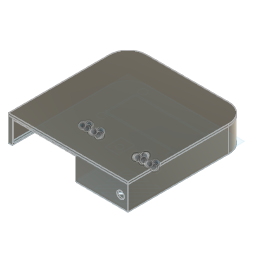
Controlador modelo 3d (sujeto a cambios) (Autodesk Fusion 360 design; units mm, degrees)
Autodesk Fusion 360 part; units mm, degrees
note: some values were not read from the file. Chosen so that the rebuilt part matches the saved one: which sketch regions a step uses; that a step has no effect; which face or edge a step refers to.
sketch "Sketch1" plane through (0, 0, 0) normal (0, 0, 1) x (1, 0, 0)
  line L0 (0, 0) -> (120, 0)
  line L1 (120, 0) -> (120, 120)
  line L2 (120, 120) -> (0, 120)
  line L3 (0, 120) -> (0, 0)
  line L4 (0, 120) -> (22, 120)
  line L5 (22, 120) -> (22, 110)
  line L6 (22, 110) -> (98, 110)
  line L7 (98, 110) -> (98, 84)
  line L8 (98, 84) -> (22, 84)
  line L9 (22, 84) -> (22, 110)
  line L10 (120, 45) -> (0, 45)
  line L11 (0, 45) -> (0, 0)
  line L12 (0, 0) -> (120, 0)
  line L13 (120, 0) -> (120, 45)
  line L14 (2, 118) -> (2, 2)
  line L15 (2, 2) -> (118, 2)
  line L16 (118, 2) -> (118, 118)
  line L17 (118, 118) -> (2, 118)
  dimension "d1" = 120
  dimension "d2" = 120
  dimension "d3" = 22
  dimension "d4" = 76
  dimension "d5" = 26
  dimension "d6" = -2
  constraint horizontal L0
  constraint vertical L1
  constraint horizontal L2
  constraint vertical L3
  constraint coincident L0.start L3.end
  constraint perpendicular L3 L4
  constraint perpendicular L4 L5
  constraint horizontal L6
  constraint vertical L7
  constraint horizontal L8
  constraint vertical L9
  constraint horizontal L10
  constraint vertical L11
  constraint horizontal L12
  constraint vertical L13
  constraint coincident L1 L10.start
  measures "d1" distance of L0.start L0.end
  measures "d2" distance of L0.start L2.end
  measures "d3" distance of L2.end L4.end
  measures "d4" distance of L5.end L6.end
  measures "d5" distance of L5.end L8.end
  measures "d43" distance of L10.end
  measures "d44" distance of L10.end
  measures "d181" distance of L10.end
  measures "d182" distance of L10.end
  measures "d201" distance of L10.end
  measures "d202" distance of L10.end
  measures "d203" distance of L10.end
sketch "Sketch2" plane through (0, 0, -50) normal (0, 0, -1) x (1, 0, 0)
  line L0 (118, -118) -> (2, -118)
  line L1 (2, -118) -> (2, -2)
  line L2 (2, -2) -> (118, -2)
  line L3 (118, -2) -> (118, -118)
  line L4 (0, 0) -> (0, -120)
  line L5 (0, -120) -> (120, -120)
  line L6 (120, -120) -> (120, 0)
  line L7 (120, 0) -> (0, 0)
  line L8 (0, 0) -> (120, 0)
  line L9 (120, 0) -> (120, -120)
  line L10 (120, -120) -> (0, -120)
  line L11 (0, -120) -> (0, 0)
  constraint horizontal L8
  constraint vertical L9
  constraint horizontal L10
  constraint vertical L11
  constraint coincident L5.end L6.start
  constraint coincident L4.start L7.end
sketch "Sketch3" plane through (120, 0, 0) normal (1, 0, 0) x (0, 1, 0)
  line L0 (120, 0) -> (0, 0)
  line L1 (0, 0) -> (0, -50)
  line L2 (0, -50) -> (120, -50)
  line L3 (120, -50) -> (120, 0)
  line L4 (0, -25) -> (50, -25)
  line L5 (50, -25) -> (50, 0)
  constraint midpoint L1 L4.start
  constraint perpendicular L1 L4
  constraint coincident L0 L5.end
  constraint perpendicular L0 L5
extrude "Extrude4" cut sketch "Sketch3" against normal blind 140 contours L0 L1 L4 L5
sketch "Sketch4" plane through (2, 0, 0) normal (1, 0, 0) x (0, 1, 0)
  line L0 (50, -2) -> (50, -25)
  line L1 (50, -25) -> (2, -25)
  line L2 (2, -25) -> (2, -48)
  line L3 (2, -48) -> (118, -48)
  line L4 (118, -48) -> (118, -2)
  line L5 (118, -2) -> (50, -2)
  line L6 (4, -27) -> (4, -46)
  line L7 (4, -46) -> (116, -46)
  line L8 (116, -46) -> (116, -4)
  line L9 (116, -4) -> (52, -4)
  line L10 (52, -4) -> (52, -27)
  line L11 (52, -27) -> (4, -27)
  line L12 (4, -27) -> (0, -27)
  line L13 (52, -4) -> (52, 0)
  dimension "d15" = -2
  constraint perpendicular L2 L12
  constraint perpendicular L5 L13
sketch "Sketch5" plane through (0, 0, 0) normal (0, 0, 1) x (-1, 0, 0)
  line L0 (-2, -50) -> (-118, -50)
  line L1 (-98, -84) -> (-22, -84)
  line L2 (-22, -84) -> (-22, -110)
  line L3 (-22, -110) -> (-98, -110)
  line L4 (-98, -110) -> (-98, -84)
  line L5 (-22, -110) -> (-98, -110)
  line L6 (-98, -110) -> (-98, -84)
  line L7 (-98, -84) -> (-22, -84)
  line L8 (-22, -84) -> (-22, -110)
  line L9 (-118, -50) -> (-118, -118)
  line L10 (-118, -118) -> (-2, -118)
  line L11 (-2, -118) -> (-2, -50)
  constraint horizontal L5
  constraint vertical L6
  constraint horizontal L7
  constraint vertical L8
  constraint coincident L1.start L4.end
  constraint coincident L2.end L3.start
sketch "Sketch6" plane through (0, 0, -1) normal (0, 0, 1) x (-1, 0, 0)
  line L0 (-22, -84) -> (-98, -84)
  line L1 (-98, -84) -> (-98, -110)
  line L2 (-98, -110) -> (-22, -110)
  line L3 (-22, -110) -> (-22, -84)
  line L4 (-22, -110) -> (-98, -110)
  line L5 (-98, -110) -> (-98, -84)
  line L6 (-98, -84) -> (-22, -84)
  line L7 (-22, -84) -> (-22, -110)
  line L8 (-35, -90) -> (-90, -90) construction
  line L9 (-90, -90) -> (-90, -105) construction
  line L10 (-90, -105) -> (-35, -105) construction
  line L11 (-35, -105) -> (-35, -90) construction
  dimension "d22" = 10
  constraint horizontal L4
  constraint vertical L5
  constraint horizontal L6
  constraint vertical L7
  constraint coincident L0.end L1.start
  constraint coincident L2.end L3.start
sketch "Sketch7" plane through (0, 0, 0) normal (0, 0, 1) x (-1, 0, 0)
  line L0 (-2, -50) -> (-118, -50)
  line L1 (-98, -84) -> (-22, -84)
  line L2 (-22, -84) -> (-22, -110)
  line L3 (-22, -110) -> (-98, -110)
  line L4 (-98, -110) -> (-98, -84)
  line L5 (-122, -120) -> (-2, -120)
  line L6 (-2, -120) -> (-2, -50)
  line L7 (-2, -50) -> (-122, -50)
  line L8 (-122, -50) -> (-122, -120)
  line L9 (-60, -79.6486) -> (-22, -79.6486)
  line L10 (-22, -79.6486) -> (-98, -79.6486)
  line L11 (-98, -79.6486) -> (-98, -69.6486)
  line L12 (-22, -69.6486) -> (-22, -79.6486)
  line L13 (-22, -79.6486) -> (-98, -79.6486)
  line L14 (-98, -79.6486) -> (-98, -67.6486)
  line L15 (-98, -67.6486) -> (-22, -67.6486)
  line L16 (-22, -67.6486) -> (-22, -79.6486)
  line L17 (-22, -79.6486) -> (-26, -79.6486)
  line L18 (-26, -79.6486) -> (-38, -79.6486)
  line L19 (-38, -67.6486) -> (-26, -67.6486)
  line L20 (-38, -67.6486) -> (-43, -67.6486)
  line L21 (-43, -67.6486) -> (-55, -67.6486)
  line L22 (-55, -79.6486) -> (-43, -79.6486)
  line L23 (-55, -67.6486) -> (-60, -67.6486)
  line L24 (-60, -67.6486) -> (-72, -67.6486)
  line L25 (-72, -79.6486) -> (-60, -79.6486)
  line L26 (-22, -79.6486) -> (-30, -79.6486)
  line L27 (-30, -79.6486) -> (-42, -79.6486)
  line L28 (-42, -79.6486) -> (-42, -67.6486)
  line L29 (-42, -67.6486) -> (-30, -67.6486)
  line L30 (-30, -67.6486) -> (-30, -79.6486)
  line L31 (-42, -67.6486) -> (-46, -67.6486)
  line L32 (-46, -67.6486) -> (-58, -67.6486)
  line L33 (-58, -67.6486) -> (-58, -79.6486)
  line L34 (-58, -79.6486) -> (-46, -79.6486)
  line L35 (-46, -79.6486) -> (-46, -67.6486)
  line L36 (-58, -79.6486) -> (-62, -79.6486)
  line L37 (-62, -79.6486) -> (-74, -79.6486)
  line L38 (-74, -79.6486) -> (-74, -67.6486)
  line L39 (-74, -67.6486) -> (-62, -67.6486)
  line L40 (-62, -67.6486) -> (-62, -79.6486)
  line L41 (-74, -67.6486) -> (-78, -67.6486)
  line L42 (-78, -67.6486) -> (-90, -67.6486)
  line L43 (-90, -67.6486) -> (-90, -79.6486)
  line L44 (-90, -79.6486) -> (-78, -79.6486)
  line L45 (-78, -79.6486) -> (-78, -67.6486)
  circle A0 centre (-36, -73.6486) radius 6
  circle A1 centre (-52, -73.6486) radius 6
  circle A2 centre (-68, -73.6486) radius 6
  circle A3 centre (-84, -73.6486) radius 6
  line L46 (-118, -50) -> (-118, -118)
  line L47 (-118, -118) -> (-2, -118)
  line L48 (-2, -118) -> (-2, -50)
  dimension "d27" = 10
  dimension "d28" = 12
  dimension "d29" = 12
  dimension "d30" = 12
  dimension "d31" = 12
  dimension "d32" = 12
  dimension "d33" = 5
  dimension "d34" = 12
  dimension "d35" = 12
  dimension "d36" = 8
  dimension "d37" = 12
  dimension "d38" = 12
  dimension "d39" = 4
  dimension "d40" = 12
  dimension "d41" = 12
  dimension "d42" = 4
  dimension "d43" = 12
  dimension "d44" = 12
  dimension "d45" = 4
  dimension "d46" = 12
  dimension "d47" = 12
  dimension "d48" = 6
  dimension "d49" = 6
  dimension "d50" = 6
  dimension "d51" = 6
  constraint horizontal L5
  constraint vertical L6
  constraint horizontal L7
  constraint vertical L8
  constraint coincident L0.start L6.end
  constraint parallel L1 L9
  constraint horizontal L10
  constraint vertical L11
  constraint vertical L12
  constraint horizontal L13
  constraint vertical L14
  constraint horizontal L15
  constraint vertical L16
  constraint coincident L9 L17.end
  constraint perpendicular L16 L17
  constraint horizontal L18
  constraint horizontal L19
  constraint coincident L15 L20.end
  constraint horizontal L21
  constraint horizontal L22
  constraint horizontal L24
  constraint horizontal L25
  constraint perpendicular L12 L26
  constraint horizontal L27
  constraint vertical L28
  constraint horizontal L29
  constraint vertical L30
  constraint perpendicular L28 L31
  constraint horizontal L32
  constraint vertical L33
  constraint horizontal L34
  constraint vertical L35
  constraint perpendicular L33 L36
  constraint horizontal L37
  constraint vertical L38
  constraint horizontal L39
  constraint vertical L40
  constraint perpendicular L38 L41
  constraint horizontal L42
  constraint vertical L43
  constraint horizontal L44
  constraint vertical L45
  constraint tangent L30 A0
  constraint tangent L15 A0
  constraint tangent L15 A1
  constraint tangent L35 A1
  constraint tangent L15 A2
  constraint tangent L40 A2
  constraint tangent L15 A3
  constraint tangent L45 A3
  measures "d27" distance of L9.end L12.start
  measures "d28" distance of L9.end L15.end
  measures "d29" distance of L17.end L18.end
  measures "d30" distance of L17.end L19.end
  measures "d31" distance of L20.end L21.end
  measures "d32" distance of L20.end L22.end
  measures "d33" distance of L21.end L23.end
  measures "d34" distance of L23.end L24.end
  measures "d35" distance of L23.end L9.start
  measures "d36" distance of L9.end L26.end
  measures "d37" distance of L26.end L27.end
  measures "d38" distance of L26.end L29.end
  measures "d39" distance of L28.end L31.end
  measures "d40" distance of L31.end L32.end
  measures "d41" distance of L31.end L34.end
  measures "d42" distance of L33.end L36.end
  measures "d43" distance of L36.end L37.end
  measures "d44" distance of L36.end L39.end
  measures "d45" distance of L38.end L41.end
  measures "d46" distance of L41.end L42.end
  measures "d47" distance of L41.end L44.end
  measures "d48" radius of A0
  measures "d49" radius of A1
  measures "d50" radius of A2
  measures "d51" radius of A3
sketch "Sketch8" plane through (0, 0, -3) normal (0, 0, -1) x (1, 0, 0)
  circle A0 centre (84, -73.6486) radius 6
  line L0 (84, -73.6486) -> (84, -67.6486)
  line L1 (84, -67.6486) -> (90, -67.6486)
  line L2 (90, -67.6486) -> (30, -67.6486)
  line L3 (30, -67.6486) -> (30, -79.6486)
  line L4 (30, -79.6486) -> (90, -79.6486)
  line L5 (90, -79.6486) -> (90, -67.6486)
  dimension "d60" = 12
  constraint coincident A0.centre L0.start
  constraint coincident A0 L0.end
  constraint vertical L0
  constraint tangent A0 L1
  constraint horizontal L2
  constraint vertical L3
  constraint horizontal L4
  constraint vertical L5
  measures "d60" distance of L1.end L4.end
sketch "Sketch9" plane through (0, 0, 0) normal (0, 0, 1) x (-1, 0, 0)
  circle A0 centre (-68, -73.6486) radius 6
  circle A1 centre (-52, -73.6486) radius 6
  circle A2 centre (-84, -73.6486) radius 6
  circle A3 centre (-36, -73.6486) radius 6
  line L0 (-2, -50) -> (-118, -50)
  line L1 (-98, -84) -> (-22, -84)
  line L2 (-22, -84) -> (-22, -110)
  line L3 (-22, -110) -> (-98, -110)
  line L4 (-98, -110) -> (-98, -84)
  line L5 (-36, -73.6486) -> (-36, -67.6486)
  line L6 (-36, -67.6486) -> (-36, -65.6486)
  line L7 (-36, -65.6486) -> (-30, -65.6486)
  line L8 (-30, -65.6486) -> (-90, -65.6486)
  line L9 (-90, -65.6486) -> (-90, -60.6486)
  line L10 (-90, -60.6486) -> (-30, -60.6486)
  line L11 (-30, -60.6486) -> (-30, -65.6486)
  line L12 (-30, -65.6486) -> (-42, -65.6486)
  line L13 (-42, -65.6486) -> (-42, -60.6486)
  line L14 (-42, -60.6486) -> (-30, -60.6486)
  line L15 (-30, -60.6486) -> (-30, -65.6486)
  line L16 (-90, -65.6486) -> (-78, -65.6486)
  line L17 (-78, -65.6486) -> (-78, -60.6486)
  line L18 (-78, -60.6486) -> (-90, -60.6486)
  line L19 (-90, -60.6486) -> (-90, -65.6486)
  line L20 (-78, -65.6486) -> (-74, -65.6486)
  line L21 (-42, -65.6486) -> (-46, -65.6486)
  line L22 (-46, -65.6486) -> (-58, -65.6486)
  line L23 (-58, -65.6486) -> (-58, -60.6486)
  line L24 (-58, -60.6486) -> (-46, -60.6486)
  line L25 (-46, -60.6486) -> (-46, -65.6486)
  line L26 (-74, -65.6486) -> (-62, -65.6486)
  line L27 (-62, -65.6486) -> (-62, -60.6486)
  line L28 (-62, -60.6486) -> (-74, -60.6486)
  line L29 (-74, -60.6486) -> (-74, -65.6486)
  line L30 (-36, -65.6486) -> (-33, -65.6486)
  line L31 (-33.5, -69.1486) -> (-33.5, -57.1486) construction
  line L32 (-33.5, -57.1486) -> (-38.5, -57.1486) construction
  line L33 (-38.5, -57.1486) -> (-38.5, -69.1486) construction
  line L34 (-38.5, -69.1486) -> (-33.5, -69.1486) construction
  line L35 (-55.1376, -57.1486) -> (-55.1376, -69.1486) construction
  line L36 (-55.1376, -69.1486) -> (-50.1376, -69.1486) construction
  line L37 (-50.1376, -69.1486) -> (-50.1376, -57.1486) construction
  line L38 (-50.1376, -57.1486) -> (-55.1376, -57.1486) construction
  line L39 (-62.3188, -60.3674) -> (-74.3188, -60.3674) construction
  line L40 (-74.3188, -60.3674) -> (-74.3188, -65.3674) construction
  line L41 (-74.3188, -65.3674) -> (-62.3188, -65.3674) construction
  line L42 (-62.3188, -65.3674) -> (-62.3188, -60.3674) construction
  line L43 (-90.3188, -65.9674) -> (-78.3188, -65.9674) construction
  line L44 (-78.3188, -65.9674) -> (-78.3188, -60.9674) construction
  line L45 (-78.3188, -60.9674) -> (-90.3188, -60.9674) construction
  line L46 (-90.3188, -60.9674) -> (-90.3188, -65.9674) construction
  line L47 (-118, -50) -> (-118, -118)
  line L48 (-118, -118) -> (-2, -118)
  line L49 (-2, -118) -> (-2, -50)
  dimension "d63" = 2
  dimension "d64" = 6
  dimension "d65" = 60
  dimension "d66" = 5
  dimension "d67" = 12
  dimension "d68" = 5
  dimension "d69" = 12
  dimension "d70" = 4
  dimension "d71" = 4
  dimension "d72" = 12
  dimension "d73" = 12
  dimension "d74" = 6
  dimension "d75" = 6
  dimension "d76" = 6
  dimension "d77" = 6
  constraint coincident A3.centre L5.start
  constraint coincident A3 L5.end
  constraint vertical L5
  constraint parallel L5 L6
  constraint perpendicular L6 L7
  constraint horizontal L8
  constraint vertical L9
  constraint horizontal L10
  constraint vertical L11
  constraint horizontal L12
  constraint vertical L13
  constraint horizontal L14
  constraint vertical L15
  constraint horizontal L16
  constraint vertical L17
  constraint horizontal L18
  constraint vertical L19
  constraint perpendicular L17 L20
  constraint perpendicular L13 L21
  constraint horizontal L22
  constraint vertical L23
  constraint horizontal L24
  constraint vertical L25
  constraint horizontal L26
  constraint vertical L27
  constraint horizontal L28
  constraint vertical L29
  constraint midpoint L7 L30.end
  measures "d63" distance of L5.end L6.end
  measures "d64" distance of L6.end L7.end
  measures "d65" distance of L7.end L8.end
  measures "d66" distance of L7.end L10.end
  measures "d67" distance of L7.end L12.end
  measures "d68" distance of L7.end L10.end
  measures "d69" distance of L8.end L16.end
  measures "d70" distance of L16.end L20.end
  measures "d71" distance of L12.end L21.end
  measures "d72" distance of L21.end L22.end
  measures "d73" distance of L20.end L26.end
extrude "Extrude16" [no effect]
sketch "Sketch10" plane through (0, 0, -25) normal (0, 0, 1) x (-1, 0, 0)
  line L0 (-119, -50) -> (-117, -50)
  line L1 (-2, -48) -> (-2, -2)
  line L2 (-118, -2) -> (-118, -48)
  line L3 (-2, -2) -> (-2, 0)
  line L4 (-2, 0) -> (-2, -50)
  line L5 (-118, -2) -> (-118, 0)
  line L6 (-173, -50) -> (-133, -50)
  line L7 (-134, -30) -> (-173, -30)
  line L8 (-173, -30) -> (-173, -50)
  line L9 (-173, -30) -> (-168, -30)
  line L10 (-168, -30) -> (-158, -30)
  line L11 (-158, -30) -> (-158, -50)
  line L12 (-158, -50) -> (-168, -50)
  line L13 (-168, -50) -> (-168, -30)
  line L14 (-158, -30) -> (-156, -30)
  line L15 (-156, -30) -> (-146, -30)
  line L16 (-146, -30) -> (-146, -50)
  line L17 (-146, -50) -> (-156, -50)
  line L18 (-156, -50) -> (-156, -30)
  line L19 (-146, -30) -> (-144, -30)
  line L20 (-144, -30) -> (-134, -30)
  line L21 (-134, -30) -> (-134, -50)
  line L22 (-134, -50) -> (-144, -50)
  line L23 (-144, -50) -> (-144, -30)
  line L24 (-134, -50) -> (-128, -50)
  line L25 (-128, -50) -> (-120, -50)
  line L26 (-120, -50) -> (-120, -40)
  line L27 (-120, -40) -> (-128, -40)
  line L28 (-128, -40) -> (-128, -50)
  line L29 (-120, -50) -> (-118, -50)
  line L30 (-118, -50) -> (-110, -50)
  line L31 (-110, -50) -> (-110, -40)
  line L32 (-110, -40) -> (-118, -40)
  line L33 (-118, -40) -> (-118, -50)
  line L34 (-110, -50) -> (-108, -50)
  line L35 (-108, -50) -> (-100, -50)
  line L36 (-100, -50) -> (-100, -40)
  line L37 (-100, -40) -> (-108, -40)
  line L38 (-108, -40) -> (-108, -50)
  line L39 (-100, -50) -> (-98, -50)
  line L40 (-98, -50) -> (-90, -50)
  line L41 (-90, -50) -> (-90, -40)
  line L42 (-90, -40) -> (-98, -40)
  line L43 (-98, -40) -> (-98, -50)
  line L44 (-90, -50) -> (-88, -50)
  line L45 (-88, -50) -> (-80, -50)
  line L46 (-80, -50) -> (-80, -40)
  line L47 (-80, -40) -> (-88, -40)
  line L48 (-88, -40) -> (-88, -50)
  line L49 (-80, -50) -> (-78, -50)
  line L50 (-78, -50) -> (-70, -50)
  line L51 (-70, -50) -> (-70, -40)
  line L52 (-70, -40) -> (-78, -40)
  line L53 (-78, -40) -> (-78, -50)
  line L54 (-70, -50) -> (-68, -50)
  line L55 (-68, -50) -> (-62, -50)
  line L56 (-62, -50) -> (-62, -44)
  line L57 (-62, -44) -> (-68, -44)
  line L58 (-68, -44) -> (-68, -50)
  line L59 (-118, -48) -> (-118, -50)
  line L60 (-117, -2) -> (-119, -2)
  line L61 (-119, -2) -> (-119, -50)
  line L62 (-117, -50) -> (-117, -2)
  dimension "d85" = 5
  dimension "d86" = 10
  dimension "d87" = 8
  dimension "d88" = 2
  constraint coincident L0 L4.end
  constraint perpendicular L0 L4
  constraint horizontal L6
  constraint horizontal L7
  constraint vertical L8
  constraint coincident L0 L6.start
  constraint perpendicular L8 L9
  constraint horizontal L10
  constraint vertical L11
  constraint horizontal L12
  constraint vertical L13
  constraint coincident L6 L11.end
  constraint coincident L7 L14.end
  constraint horizontal L15
  constraint vertical L16
  constraint horizontal L17
  constraint vertical L18
  constraint coincident L6 L16.end
  constraint coincident L7 L19.end
  constraint horizontal L20
  constraint vertical L21
  constraint horizontal L22
  constraint vertical L23
  constraint coincident L0 L24.end
  constraint horizontal L25
  constraint vertical L26
  constraint horizontal L27
  constraint vertical L28
  constraint midpoint L0 L29.end
  constraint horizontal L30
  constraint vertical L31
  constraint horizontal L32
  constraint vertical L33
  constraint coincident L0 L34.end
  constraint perpendicular L31 L34
  constraint horizontal L35
  constraint vertical L36
  constraint horizontal L37
  constraint vertical L38
  constraint coincident L0 L39.end
  constraint perpendicular L36 L39
  constraint horizontal L40
  constraint vertical L41
  constraint horizontal L42
  constraint vertical L43
  constraint perpendicular L41 L44
  constraint horizontal L45
  constraint vertical L46
  constraint horizontal L47
  constraint vertical L48
  constraint coincident L0 L49.end
  constraint perpendicular L46 L49
  constraint horizontal L50
  constraint vertical L51
  constraint horizontal L52
  constraint vertical L53
  constraint coincident L0 L54.end
  constraint perpendicular L51 L54
  constraint horizontal L55
  constraint vertical L56
  constraint horizontal L57
  constraint vertical L58
  constraint coincident L0 L29.end
  constraint perpendicular L0 L59
  measures "d85" distance of L7.end L9.end
  measures "d86" distance of L19.end L7.start
  measures "d87" distance of L29.end L30.end
  measures "d88" distance of L40.end L44.end
sketch "Sketch11" plane through (0, 50, 0) normal (0, 1, 0) x (-1, 0, 0)
  line L0 (-110, -25) -> (-100, -25)
  line L1 (-100, -25) -> (-100, -15)
  line L2 (-100, -15) -> (-110, -15)
  line L3 (-110, -15) -> (-110, -25)
  line L4 (-110, -15) -> (-4, -15)
  line L5 (-4, -15) -> (-4, -25)
  line L6 (-4, -25) -> (-110, -25)
  line L7 (-110, -25) -> (-110, -15)
  constraint horizontal L4
  constraint vertical L5
  constraint horizontal L6
  constraint vertical L7
  constraint coincident L2.end L3.start
sketch "Sketch12" plane through (0, 0, 0) normal (0, 0, 1) x (-1, 0, 0)
  line L0 (-118, -2) -> (-234, -2)
  line L1 (-234, -2) -> (-234, 48)
  line L2 (-234, 48) -> (-118, 48)
  line L3 (-118, 48) -> (-118, -2)
  line L4 (-118, 0) -> (-2, 0)
  line L5 (-2, 0) -> (-2, -2)
  line L6 (-2, -2) -> (-118, -2)
  line L7 (-118, -2) -> (-118, 0)
  line L8 (-118, -2) -> (-119, -2)
  line L9 (-119, -2) -> (-119, -50)
  line L10 (-118, -50) -> (-118, -2)
  line L11 (-119, -50) -> (-118, -50)
  dimension "d95" = 2
  constraint horizontal L0
  constraint vertical L1
  constraint horizontal L2
  constraint vertical L3
  constraint coincident L0.start L3.end
  constraint horizontal L4
  constraint vertical L5
  constraint horizontal L6
  constraint vertical L7
  measures "d95" distance of L4.start L0.start
extrude "Extrude25" [no effect]
sketch "Sketch13" plane through (0, 0, 0) normal (1, 0, 0) x (0, 1, 0)
  line L0 (42, -15) -> (40, -17)
  line L1 (42, -15) -> (40, -15)
  line L2 (40, -15) -> (40, -17)
  constraint horizontal L1
  constraint perpendicular L1 L2
extrude "Extrude26" cut sketch "Sketch13" along normal blind 115
sketch "Sketch14" plane through (0, 40, 0) normal (0, -1, 0) x (1, 0, 0)
  line L0 (10, -17) -> (4, -17)
  line L1 (4, -17) -> (4, -25)
  line L2 (4, -25) -> (10, -25)
  line L3 (10, -25) -> (10, -17)
  line L4 (5, -18) -> (9, -18)
  line L5 (9, -18) -> (9, -24)
  line L6 (9, -24) -> (5, -24)
  line L7 (5, -24) -> (5, -18)
  line L8 (13, -18) -> (19, -18)
  line L9 (19, -18) -> (19, -24)
  line L10 (19, -24) -> (13, -24)
  line L11 (13, -24) -> (13, -18)
  line L12 (23, -18) -> (29, -18)
  line L13 (29, -18) -> (29, -24)
  line L14 (29, -24) -> (23, -24)
  line L15 (23, -24) -> (23, -18)
  line L16 (33, -18) -> (39, -18)
  line L17 (39, -18) -> (39, -24)
  line L18 (39, -24) -> (33, -24)
  line L19 (33, -24) -> (33, -18)
  line L20 (43, -18) -> (49, -18)
  line L21 (49, -18) -> (49, -24)
  line L22 (49, -24) -> (43, -24)
  line L23 (43, -24) -> (43, -18)
  line L24 (53, -18) -> (59, -18)
  line L25 (59, -18) -> (59, -24)
  line L26 (59, -24) -> (53, -24)
  line L27 (53, -24) -> (53, -18)
  line L28 (63, -18) -> (69, -18)
  line L29 (69, -18) -> (69, -24)
  line L30 (69, -24) -> (63, -24)
  line L31 (63, -24) -> (63, -18)
  line L32 (77, -18) -> (85, -18)
  line L33 (85, -18) -> (85, -24)
  line L34 (85, -24) -> (77, -24)
  line L35 (77, -24) -> (77, -18)
  line L36 (89, -18) -> (97, -18)
  line L37 (97, -18) -> (97, -24)
  line L38 (97, -24) -> (89, -24)
  line L39 (89, -24) -> (89, -18)
  line L40 (101, -18) -> (109, -18)
  line L41 (109, -18) -> (109, -24)
  line L42 (109, -24) -> (101, -24)
  line L43 (101, -24) -> (101, -18)
  constraint horizontal L4
  constraint vertical L5
  constraint horizontal L6
  constraint vertical L7
  constraint horizontal L8
  constraint vertical L9
  constraint horizontal L10
  constraint vertical L11
  constraint horizontal L12
  constraint vertical L13
  constraint horizontal L14
  constraint vertical L15
  constraint horizontal L16
  constraint vertical L17
  constraint horizontal L18
  constraint vertical L19
  constraint horizontal L20
  constraint vertical L21
  constraint horizontal L22
  constraint vertical L23
  constraint horizontal L24
  constraint vertical L25
  constraint horizontal L26
  constraint vertical L27
  constraint horizontal L28
  constraint vertical L29
  constraint horizontal L30
  constraint vertical L31
  constraint horizontal L32
  constraint vertical L33
  constraint horizontal L34
  constraint vertical L35
  constraint horizontal L36
  constraint vertical L37
  constraint horizontal L38
  constraint vertical L39
  constraint horizontal L40
  constraint vertical L41
  constraint horizontal L42
  constraint vertical L43
extrude "Extrude27" cut sketch "Sketch14" against normal blind 10 contours L4 L5 L6 L7 | L8 L9 L10 L11 | L12 L13 L14 L15 | L16 L17 L18 L19 | L20 L21 L22 L23 | L24 L25 L26 L27 | L28 L29 L30 L31 | L32 L33 L34 L35 | L36 L37 L38 L39 | L40 L41 L42 L43
sketch "Sketch15" plane through (0, 0, -15) normal (0, 0, 1) x (-1, 0, 0)
  line L0 (-4, -50) -> (-110, -50)
  line L1 (-110, -50) -> (-110, -54)
  line L2 (-110, -54) -> (-4, -54)
  line L3 (-4, -54) -> (-4, -50)
  circle A0 centre (-7, -45) radius 2
  circle A1 centre (-16, -45) radius 2
  circle A2 centre (-26, -45) radius 2
  circle A3 centre (-36, -45) radius 2
  circle A4 centre (-46, -45) radius 2
  circle A5 centre (-56, -45) radius 2
  circle A6 centre (-66, -45) radius 2
  circle A7 centre (-81, -45) radius 2
  circle A8 centre (-93, -45) radius 2
  circle A9 centre (-105, -45) radius 2
extrude "Extrude28" cut sketch "Sketch15" against normal blind 2 contours A0 | A1 | A2 | A3 | A4 | A5 | A6 | A7 | A8 | A9
sketch "Sketch16" plane through (0, 0, -17) normal (0, 0, 1) x (-1, 0, 0)
  circle A0 centre (-105, -45) radius 1.7589
  line L0 (-104.8, -45.2) -> (-104.8, -46.7475)
  line L1 (-104.8, -44.8) -> (-104.8, -43.2525)
  line L2 (-105.2, -45.2) -> (-105.2, -46.7475)
  line L3 (-105.2, -44.8) -> (-105.2, -43.2525)
  line L4 (-105.2, -45.2) -> (-106.7475, -45.2)
  line L5 (-105.2, -44.8) -> (-106.7475, -44.8)
  line L6 (-104.8, -45.2) -> (-103.2525, -45.2)
  line L7 (-105.2, -43.2525) -> (-105.2, -44.8)
  line L8 (-105.2, -45.2) -> (-105.2, -46.7475)
  line L9 (-106.7589, -44.8) -> (-105.2, -44.8)
  line L10 (-104.8, -44.8) -> (-103.2525, -44.8)
  line L11 (-104.8, -46.7475) -> (-104.8, -45.2)
  line L12 (-104.8, -44.8) -> (-104.8, -43.2525)
  line L13 (-8.7321, -44) -> (-5.2679, -44)
  arc A1 (-5.2679, -44) -> (-8.7321, -44) centre (-7, -45) ccw
  constraint vertical L11
  constraint vertical L7
  constraint horizontal L9
  constraint collinear L7 L8
  constraint collinear L9 L10
  constraint collinear L11 L12
  constraint coincident A0 L4.end
  constraint coincident A0 L5.end
  constraint coincident A0 L3.end
  constraint coincident A0 L1.end
  constraint coincident A0 L10.end
  constraint coincident A0 L6.end
  constraint coincident A0 L0.end
  constraint coincident A0 L2.end
sketch "Sketch17" plane through (0, 0, 0) normal (0, 0, 1) x (1, 0, 0)
  line L0 (0, 0) -> (98, 0)
  line L1 (98, 0) -> (98, 40)
  line L2 (98, 40) -> (0, 40)
  line L3 (0, 40) -> (0, 0)
  line L4 (0, 0) -> (0, -30)
  circle A0 centre (4, -30) radius 4
  circle A1 centre (49, -30) radius 4
  circle A2 centre (94, -30) radius 4
  circle A3 centre (49, -30) radius 4
  circle A4 centre (4, -30) radius 4
  line L5 (0, 0) -> (0, -30)
  circle A5 centre (94, -30) radius 4
  line L6 (0, -30) -> (98, -30)
  line L7 (26.5, -30) -> (19.5, -30)
  line L8 (71.5, -30) -> (78.5, -30)
  circle A6 centre (19.5, -30) radius 4
  circle A7 centre (78.5, -30) radius 4
  circle A8 centre (49, -30) radius 15
  line L9 (-30, 60) -> (128, 60)
  line L10 (128, 60) -> (128, -70)
  line L11 (128, -70) -> (-30, -70)
  line L12 (-30, -70) -> (-30, 60)
  line L13 (-30, -70) -> (128, -70)
  line L14 (128, -70) -> (128, -100)
  line L15 (128, -100) -> (-30, -100)
  line L16 (-30, -100) -> (-30, -70)
  line L17 (-30, 60) -> (128, 60)
  line L18 (128, 60) -> (128, -100)
  line L19 (128, -100) -> (-30, -100)
  line L20 (-30, -100) -> (-30, 60)
  line L21 (-25, -100) -> (-25, -95)
  line L22 (-25, -95) -> (-25, -70)
  line L23 (-25, -70) -> (-25, -100)
  line L24 (-25, -70) -> (30, -70)
  line L25 (-25, -70) -> (50, -70)
  line L26 (-25, -70) -> (70, -70)
  line L27 (-25, -70) -> (60, -70)
  line L28 (60, -70) -> (60, -100)
  dimension "d130" = 98
  dimension "d131" = 40
  dimension "d132" = 8
  dimension "d135" = 90
  dimension "d136" = 0
  dimension "d139" = 90
  dimension "d140" = 0
  dimension "d141" = 8
  dimension "d142" = 7
  dimension "d143" = 7
  dimension "d144" = 8
  dimension "d145" = 8
  dimension "d146" = 30
  dimension "d147" = 158
  dimension "d148" = 158
  dimension "d149" = 30
  dimension "d150" = 55
  dimension "d151" = 75
  dimension "d152" = 85
  dimension "d153" = 160
  dimension "d154" = 158
  constraint horizontal L0
  constraint vertical L1
  constraint horizontal L2
  constraint vertical L3
  constraint coincident L0.start L3.end
  constraint perpendicular L0 L4
  constraint coincident L4.end A0
  constraint coincident L4.end A4
  constraint coincident A2 L6.end
  constraint perpendicular L5 L6
  constraint parallel L6 L7
  constraint parallel L6 L8
  constraint coincident L7.end A6.centre
  constraint coincident L8.end A7.centre
  constraint concentric A1 A8
  constraint horizontal L9
  constraint vertical L10
  constraint horizontal L11
  constraint vertical L12
  constraint horizontal L13
  constraint vertical L14
  constraint horizontal L15
  constraint vertical L16
  constraint horizontal L17
  constraint vertical L18
  constraint horizontal L19
  constraint vertical L20
  constraint coincident L15 L21.start
  constraint perpendicular L15 L21
  constraint coincident L11 L22.end
  constraint perpendicular L11 L22
  constraint perpendicular L22 L24
  constraint perpendicular L22 L25
  constraint coincident L13 L26.end
  constraint perpendicular L22 L27
  constraint coincident L15 L28.end
  constraint perpendicular L15 L28
  measures "d130" distance of L0.start L0.end
  measures "d131" distance of L0.start L2.end
  measures "d132" diameter of A0
  measures "d141" diameter of A4
  measures "d142" distance of L7.start L7.end
  measures "d143" distance of L8.start L8.end
  measures "d144" diameter of A6
  measures "d145" diameter of A7
  measures "d146" diameter of A8
  measures "d147" distance of L9.start L9.end
  measures "d148" distance of L11.end L10.end
  measures "d149" distance of L11.end L15.end
  measures "d150" distance of L22.end L24.end
  measures "d151" distance of L22.end L25.end
  measures "d152" distance of L22.end L27.end
  measures "d153" distance of L9.start L15.end
  measures "d154" distance of L14.end L15.end
sketch "Sketch18" plane through (0, 0, 0) normal (0, 0, 1) x (1, 0, 0)
  line L0 (-30, 60) -> (130, 60)
  line L1 (130, 60) -> (130, -100)
  line L2 (130, -100) -> (-30, -100)
  line L3 (-30, -100) -> (-30, 60)
  line L4 (128, -98) -> (-28, -98)
  line L5 (-28, -98) -> (-28, 58)
  line L6 (-28, 58) -> (128, 58)
  line L7 (128, 58) -> (128, -98)
  dimension "d155" = 2
  constraint horizontal L0
  constraint vertical L1
  constraint horizontal L2
  constraint vertical L3
extrude "Extrude32" add sketch "Sketch18" along normal blind 2 separate body contours L4 L5 L6 L7 makes body 1
extrude "Extrude33" add sketch "Sketch18" along normal blind 32 bodies 1
extrude "Extrude34" cut sketch "Sketch17" along normal blind 30 contours L0 L1 L2 L3 | A0 A4 L6 | A0 A4 L6 | A1 A3 L6 | A1 A3 L6 | A2 A5 L6 | A2 A5 L6 | L6 L7 A6 | L6 L7 A6 | L6 L8 A7 | L6 L8 A7 | L11 L13 L15 L19 L21 L22 L23 L24 L25 L26 L27 L28 bodies 1
sketch "Sketch19" plane through (0, 0, 2) normal (0, 0, 1) x (-1, 0, 0)
  line L0 (-60, 70) -> (-60, 98)
  line L1 (-60, 98) -> (-128, 98)
  line L2 (-128, 98) -> (-128, -58)
  line L3 (-128, -58) -> (28, -58)
  line L4 (28, -58) -> (28, 98)
  line L5 (28, 98) -> (25, 98)
  line L6 (25, 98) -> (25, 70)
  line L7 (25, 70) -> (-60, 70)
  line L8 (0, -40) -> (-98, -40)
  line L9 (-98, -40) -> (-98, 0)
  line L10 (-98, 0) -> (0, 0)
  line L11 (0, 0) -> (0, -40)
  circle A0 centre (-4, 30) radius 4
  circle A1 centre (-94, 30) radius 4
  circle A2 centre (-49, 30) radius 4
  circle A3 centre (-19.5, 30) radius 4
  circle A4 centre (-78.5, 30) radius 4
  circle A5 centre (-2.5, -47.5) radius 2.5
  arc A6 (-95.5, -50) -> (-95.5, -45) centre (-95.5, -47.5) ccw
  circle A7 centre (-95.5, -47.5) radius 2.5
  circle A8 centre (-95.5, -47.5) radius 5
  arc A9 (-98, 7.5) -> (-95.5, 10) centre (-95.5, 7.5) ccw
  circle A10 centre (-95.5, 7.5) radius 2.5
  arc A11 (-2.5, 10) -> (-2.5, 5) centre (-2.5, 7.5) ccw
  circle A12 centre (-2.5, 7.5) radius 2.5
  circle A13 centre (-2.5, 7.5) radius 5
  circle A14 centre (-95.5, 7.5) radius 5
  circle A15 centre (-2.5, -47.5) radius 5
  dimension "d165" = 10
  dimension "d166" = 10
  dimension "d167" = 10
  dimension "d168" = 10
  constraint concentric A6 A7
  constraint coincident A6.end A7
  constraint concentric A6 A8
  constraint concentric A9 A10
  constraint coincident A9.end A10
  constraint concentric A11 A12
  constraint coincident A11.end A12
  constraint concentric A11 A13
  constraint concentric A9 A14
  constraint concentric A5 A15
  measures "d165" diameter of A8
  measures "d166" diameter of A13
  measures "d167" diameter of A14
  measures "d168" diameter of A15
extrude "Extrude35" add sketch "Sketch19" along normal blind 8 contours A8 | A13 | A14 | A15 bodies 1
sketch "Sketch20" plane through (0, 0, 2) normal (0, 0, 1) x (-1, 0, 0)
  circle A0 centre (-2.5, -47.5) radius 5
  circle A1 centre (-95.5, -47.5) radius 5
  line L0 (-60, 70) -> (-60, 98)
  line L1 (-60, 98) -> (-128, 98)
  line L2 (-128, 98) -> (-128, -58)
  line L3 (-128, -58) -> (28, -58)
  line L4 (28, -58) -> (28, 98)
  line L5 (28, 98) -> (25, 98)
  line L6 (25, 98) -> (25, 70)
  line L7 (25, 70) -> (-60, 70)
  line L8 (0, -40) -> (-98, -40)
  line L9 (-98, -40) -> (-98, 0)
  line L10 (-98, 0) -> (0, 0)
  line L11 (0, 0) -> (0, -40)
  circle A2 centre (-4, 30) radius 4
  circle A3 centre (-94, 30) radius 4
  circle A4 centre (-49, 30) radius 4
  circle A5 centre (-19.5, 30) radius 4
  circle A6 centre (-78.5, 30) radius 4
  circle A7 centre (-95.5, 7.5) radius 5
  circle A8 centre (-2.5, 7.5) radius 5
  line L12 (-49, 20) -> (-57, 20)
  line L13 (-57, 20) -> (-41, 20)
  line L14 (-41, 46) -> (-57, 46)
  line L15 (-49, 20) -> (-41, 20)
  line L16 (-41, 20) -> (-41, 46)
  line L17 (-41, 20) -> (-59, 20)
  line L18 (-59, 20) -> (-59, 46)
  line L19 (-59, 46) -> (-41, 46)
  line L20 (-41, 46) -> (-41, 20)
  line L21 (-49, 22) -> (-43, 22)
  line L22 (-43, 22) -> (-49, 22)
  line L23 (-55, 24) -> (-55, 36)
  line L24 (-55, 36) -> (-43, 36)
  line L25 (-43, 36) -> (-43, 24)
  line L26 (-43, 24) -> (-55, 24)
  line L27 (-55, 24) -> (-55, 36)
  line L28 (-43, 22) -> (-55, 22)
  line L29 (-55, 22) -> (-55, 38)
  line L30 (-55, 38) -> (-43, 38)
  line L31 (-43, 38) -> (-43, 22)
  line L32 (-55, 22) -> (-55, 20)
  line L33 (-55, 20) -> (-57, 20)
  line L34 (-57, 20) -> (-57, 23)
  line L35 (-55, 38) -> (-55, 46)
  line L36 (-57, 46) -> (-57, 41)
  circle A9 centre (-57, 39) radius 2
  circle A10 centre (-57, 25) radius 2
  line L37 (-41, 46) -> (-59, 46)
  line L38 (-59, 46) -> (-59, 42)
  line L39 (-59, 42) -> (-41, 42)
  line L40 (-41, 42) -> (-41, 46)
  dimension "d173" = 10
  dimension "d174" = 8
  dimension "d176" = 26
  dimension "d177" = 18
  dimension "d178" = 6
  dimension "d181" = 12
  dimension "d182" = 12
  dimension "d183" = 3
  dimension "d184" = 5
  dimension "d185" = 4
  constraint horizontal L13
  constraint horizontal L14
  constraint perpendicular L14 L16
  constraint horizontal L17
  constraint vertical L18
  constraint horizontal L19
  constraint vertical L20
  constraint perpendicular L16 L21
  constraint parallel L21 L22
  constraint horizontal L24
  constraint vertical L25
  constraint horizontal L26
  constraint vertical L27
  constraint horizontal L28
  constraint vertical L29
  constraint horizontal L30
  constraint vertical L31
  constraint coincident L13 L32.end
  constraint coincident L12 L32.end
  constraint perpendicular L13 L34
  constraint coincident L19 L35.end
  constraint coincident L14 L35.end
  constraint perpendicular L14 L36
  constraint coincident L36.end A9
  constraint coincident L34.end A10
  constraint horizontal L37
  constraint vertical L38
  constraint horizontal L39
  constraint vertical L40
  measures "d173" distance of A4.centre L12.start
  measures "d174" distance of L12.start L12.end
  measures "d176" distance of L12.end L14.end
  measures "d177" distance of L13.end L17.end
  measures "d178" distance of L21.start L21.end
  measures "d181" distance of L23.start L23.end
  measures "d182" distance of L23.end L23.start
  measures "d183" distance of L12.end L34.end
  measures "d184" distance of L14.end L36.end
  measures "d185" distance of L14.start L39.end
sketch "Sketch21" plane through (0, 0, 2) normal (0, 0, 1) x (-1, 0, 0)
  line L0 (-41, 46) -> (-59, 46)
  line L1 (-59, 46) -> (-59, 42)
  line L2 (-59, 42) -> (-41, 42)
  line L3 (-41, 42) -> (-41, 46)
  constraint horizontal L0
  constraint vertical L1
  constraint horizontal L2
  constraint vertical L3
extrude "Extrude36" add sketch "Sketch20" along normal blind 5 contours L12 L13 L15 L16 L17 L20 L21 L22 L25 L28 L30 L31 L32 L35 L39 | L12 L13 L17 L23 L27 L29 L32 L33 L34 A10 | L17 L18 L34 A10 | A10 | L35 L36 A9 L39 | L18 L23 L27 L29 L35 A9 A10 | A9 | L18 L36 A9 L39 bodies 1
sketch "Sketch22" plane through (0, 0, 2) normal (0, 0, 1) x (-1, 0, 0)
  circle A0 centre (-2.5, 7.5) radius 5
  circle A1 centre (-95.5, 7.5) radius 5
  circle A2 centre (-78.5, 30) radius 4
  circle A3 centre (-19.5, 30) radius 4
  circle A4 centre (-94, 30) radius 4
  circle A5 centre (-4, 30) radius 4
  line L0 (0, -40) -> (-98, -40)
  line L1 (-98, -40) -> (-98, 0)
  line L2 (-98, 0) -> (0, 0)
  line L3 (0, 0) -> (0, -40)
  line L4 (-60, 70) -> (-60, 98)
  line L5 (-60, 98) -> (-128, 98)
  line L6 (-128, 98) -> (-128, -58)
  line L7 (-128, -58) -> (28, -58)
  line L8 (28, -58) -> (28, 98)
  line L9 (28, 98) -> (25, 98)
  line L10 (25, 98) -> (25, 70)
  line L11 (25, 70) -> (-60, 70)
  circle A6 centre (-95.5, -47.5) radius 5
  circle A7 centre (-2.5, -47.5) radius 5
  line L12 (-59, 42) -> (-41, 42)
  line L13 (-41, 42) -> (-41, 20)
  line L14 (-41, 20) -> (-55, 20)
  line L15 (-55, 20) -> (-57, 20)
  line L16 (-57, 20) -> (-59, 20)
  line L17 (-59, 20) -> (-59, 42)
  circle A8 centre (-4, 30) radius 6
  circle A9 centre (-19.5, 30) radius 6
  circle A10 centre (-78.5, 30) radius 6
  circle A11 centre (-94, 30) radius 6
  line L18 (-3, 24.0839) -> (-3, 26.127)
  line L19 (-5, 26.127) -> (-5, 24.0839)
  line L20 (-0.1459, 31.0705) -> (1.6235, 32.092)
  line L21 (0.6235, 33.8241) -> (-1.1459, 32.8025)
  line L22 (-6.8541, 32.8025) -> (-8.6235, 33.8241)
  line L23 (-9.6235, 32.092) -> (-7.8541, 31.0705)
  line L24 (-19.5, 24) -> (-18.5, 24)
  line L25 (-18.5, 24) -> (-20.5, 24)
  line L26 (-18.5, 24) -> (-18.5, 26.127)
  line L27 (-20.5, 24) -> (-20.5, 26.127)
  line L28 (-25.1962, 32.134) -> (-23.3541, 31.0705)
  line L29 (-24.1962, 33.866) -> (-22.3541, 32.8025)
  line L30 (-14.8038, 33.866) -> (-16.6459, 32.8025)
  line L31 (-13.8038, 32.134) -> (-15.6459, 31.0705)
  line L32 (-78.5, 24) -> (-77.5, 24)
  line L33 (-77.5, 24) -> (-78.5, 24)
  line L34 (-77.5, 24) -> (-78.5, 24)
  line L35 (-77.5, 24) -> (-79.5, 24)
  line L36 (-73.8038, 33.866) -> (-75.6459, 32.8025)
  line L37 (-83.1962, 33.866) -> (-81.3541, 32.8025)
  line L38 (-84.1962, 32.134) -> (-82.3541, 31.0705)
  line L39 (-79.5, 24) -> (-79.5, 26.127)
  line L40 (-77.5, 24) -> (-77.5, 26.127)
  line L41 (-72.8038, 32.134) -> (-74.6459, 31.0705)
  line L42 (-94, 24) -> (-93, 24)
  line L43 (-93, 24) -> (-95, 24)
  line L44 (-88.3038, 32.134) -> (-90.1459, 31.0705)
  line L45 (-91.1459, 32.8025) -> (-89.3038, 33.866)
  line L46 (-98.6962, 33.866) -> (-96.8541, 32.8025)
  line L47 (-95, 24) -> (-95, 26.127)
  line L48 (-97.8541, 31.0705) -> (-99.6962, 32.134)
  line L49 (-93, 26.127) -> (-93, 24)
  dimension "d188" = 12
  dimension "d189" = 12
  dimension "d190" = 12
  dimension "d191" = 12
  dimension "d196" = 1
  dimension "d197" = 2
  dimension "d200" = 1
  dimension "d201" = 1
  dimension "d202" = 1
  dimension "d203" = 2
  dimension "d206" = 1
  constraint concentric A5 A8
  constraint concentric A3 A9
  constraint concentric A2 A10
  constraint concentric A4 A11
  constraint coincident A8 L23.start
  constraint coincident A8 L22.end
  constraint coincident A8 L19.end
  constraint coincident A8 L18.start
  constraint coincident A8 L20.end
  constraint coincident A8 L21.start
  constraint coincident A9 L24.start
  constraint perpendicular L24 L26
  constraint perpendicular L25 L27
  constraint coincident A5 L18.end
  constraint coincident A5 L19.start
  constraint coincident A5 L23.end
  constraint coincident A5 L22.start
  constraint coincident A5 L21.end
  constraint coincident A5 L20.start
  constraint coincident A3 L26.end
  constraint coincident A3 L27.end
  constraint coincident A3 L28.end
  constraint coincident A3 L29.end
  constraint coincident A3 L30.end
  constraint coincident A3 L31.end
  constraint coincident A10 L32.start
  constraint parallel L33 L34
  constraint parallel L34 L35
  constraint perpendicular L35 L39
  constraint perpendicular L34 L40
  constraint coincident A2 L39.end
  constraint coincident A2 L40.end
  constraint coincident A2 L41.end
  constraint coincident A2 L36.end
  constraint coincident A2 L37.end
  constraint coincident A2 L38.end
  constraint coincident A11 L42.start
  constraint horizontal L43
  constraint vertical L47
  constraint coincident A4 L47.end
  constraint coincident A4 L48.start
  constraint coincident A4 L49.start
  constraint coincident A4 L46.end
  constraint coincident A4 L45.start
  constraint coincident A4 L44.end
  measures "d188" diameter of A8
  measures "d189" diameter of A9
  measures "d190" diameter of A10
  measures "d191" diameter of A11
  measures "d196" distance of L24.start L24.end
  measures "d197" distance of L24.end L25.end
  measures "d200" distance of L32.start L32.end
  measures "d201" distance of L32.end L32.start
  measures "d202" distance of L32.end L32.start
  measures "d203" distance of L32.end L35.end
  measures "d206" distance of L42.start L42.end
extrude "Extrude37" add sketch "Sketch22" along normal blind 3 contours A2 A10 L40 L41 | A2 A10 L36 L41 | A2 A10 L39 L40 | A2 A10 L36 L37 | A2 A10 L38 L39 | A2 A10 L37 L38 | A3 A9 L26 L31 | A3 A9 L30 L31 | A3 A9 L26 L27 | A3 A9 L29 L30 | A3 A9 L27 L28 | A3 A9 L28 L29 | A4 A11 L44 L49 | A4 A11 L44 L45 | A4 A11 L47 L49 | A4 A11 L45 L46 | A4 A11 L47 L48 | A4 A11 L46 L48 | A5 A8 L18 L20 | A5 A8 L20 L21 | A5 A8 L18 L19 | A5 A8 L21 L22 | A5 A8 L19 L23 | A5 A8 L22 L23 bodies 1
sketch "Sketch23" plane through (0, 0, 5) normal (0, 0, 1) x (-1, 0, 0)
  circle A0 centre (-4, 30) radius 4
  circle A1 centre (-4, 30) radius 6
extrude "Extrude38" cut sketch "Sketch22" along normal blind 4 contours A2 | A2 A10 L36 L41 | A2 A10 L39 L40 | A2 A10 L37 L38 | A4 | A4 A11 L44 L45 | A4 A11 L47 L49 | A4 A11 L46 L48 bodies 1
extrude "Extrude39" cut sketch "Sketch22" along normal blind 4 contours A3 | A3 A9 L30 L31 | A3 A9 L26 L27 | A3 A9 L28 L29 | A5 | A5 A8 L20 L21 | A5 A8 L18 L19 | A5 A8 L22 L23 bodies 1
sketch "Sketch24" plane through (0, -100, 0) normal (0, -1, 0) x (1, 0, 0)
  line L0 (-25, 0) -> (-25, 30)
  line L1 (-25, 30) -> (60, 30)
  line L2 (60, 30) -> (60, 0)
  line L3 (60, 0) -> (130, 0)
  line L4 (130, 0) -> (130, 32)
  line L5 (130, 32) -> (-30, 32)
  line L6 (-30, 32) -> (-30, 0)
  line L7 (-30, 0) -> (-25, 0)
  circle A0 centre (120, 15) radius 5
extrude "Extrude40" cut sketch "Sketch24" against normal blind 26 contours A0 bodies 1
fillet "Fillet5" radius 25 4 edges at (128, 58, 17) (-28, 58, 17) (130, 60, 16) (-30, 60, 16) on bodies 1
sketch "Sketch25" plane through (0, 0, 0) normal (0, 0, -1) x (1, 0, 0)
  arc A0 (-30, -35) -> (-5, -60) centre (-5, -35) ccw
  line L0 (-5, -60) -> (105, -60)
  arc A1 (105, -60) -> (130, -35) centre (105, -35) ccw
  line L1 (130, -35) -> (130, 100)
  line L2 (130, 100) -> (60, 100)
  line L3 (60, 100) -> (60, 70)
  line L4 (60, 70) -> (-25, 70)
  line L5 (-25, 70) -> (-25, 100)
  line L6 (-25, 100) -> (-30, 100)
  line L7 (-30, 100) -> (-30, -35)
  line L8 (98, -40) -> (0, -40)
  line L9 (0, -40) -> (0, 0)
  line L10 (0, 0) -> (98, 0)
  line L11 (98, 0) -> (98, -40)
  circle A2 centre (4, 30) radius 4
  circle A3 centre (94, 30) radius 4
  circle A4 centre (49, 30) radius 4
  circle A5 centre (19.5, 30) radius 4
  circle A6 centre (78.5, 30) radius 4
  line L12 (80, 95) -> (125, 50)
  line L13 (89, 95) -> (125, 59)
  line L14 (98, 95) -> (125, 68)
  line L15 (107, 95) -> (125, 77)
  line L16 (116, 95) -> (125, 86)
  line L17 (80, 87) -> (117, 50)
  line L18 (80, 79) -> (109, 50)
  line L19 (80, 71) -> (101, 50)
  line L20 (80, 63) -> (93, 50)
  line L21 (80, 55) -> (85, 50)
  line L22 (116, 95) -> (107, 95)
  line L23 (98, 95) -> (80, 95)
  line L24 (89, 95) -> (98, 95)
  line L25 (107, 95) -> (116, 95)
  line L26 (125, 59) -> (125, 68)
  line L27 (125, 77) -> (125, 86)
  line L28 (80, 95) -> (80, 87)
  line L29 (117, 50) -> (125, 50)
  line L30 (85, 50) -> (93, 50)
  line L31 (101, 50) -> (109, 50)
  line L32 (80, 79) -> (80, 71)
  line L33 (80, 63) -> (80, 55)
  constraint horizontal L22
  constraint vertical L28
  constraint horizontal L30
  constraint vertical L26
  constraint coincident L19.end L30
  constraint coincident L17.end L30
  constraint coincident L13.start L22
  constraint coincident L14.start L22
  constraint collinear L22 L23
  constraint collinear L24 L25
  constraint collinear L26 L27
  constraint collinear L28 L32
  constraint collinear L29 L30
  constraint collinear L30 L31
  constraint collinear L32 L33
extrude "Extrude41" cut sketch "Sketch25" against normal blind 5 contours L12 L17 L28 L29 | L13 L14 L23 L24 L26 | L15 L16 L22 L25 L27 | L18 L19 L31 L32 | L20 L21 L30 L33 bodies 1
sketch "Sketch26" plane through (0, 0, 0) normal (0, 0, -1) x (1, 0, 0)
  line L0 (117, 50) -> (80, 87)
  line L1 (80, 87) -> (80, 95)
  line L2 (80, 95) -> (125, 50)
  line L3 (125, 50) -> (117, 50)
  line L4 (101, 50) -> (80, 71)
  line L5 (80, 71) -> (80, 79)
  line L6 (80, 79) -> (109, 50)
  line L7 (109, 50) -> (101, 50)
  line L8 (125, 68) -> (125, 59)
  line L9 (125, 59) -> (89, 95)
  line L10 (89, 95) -> (98, 95)
  line L11 (98, 95) -> (125, 68)
  line L12 (85, 50) -> (80, 55)
  line L13 (80, 55) -> (80, 63)
  line L14 (80, 63) -> (93, 50)
  line L15 (93, 50) -> (85, 50)
  line L16 (125, 86) -> (125, 77)
  line L17 (125, 77) -> (107, 95)
  line L18 (107, 95) -> (116, 95)
  line L19 (116, 95) -> (125, 86)
  arc A0 (-30, -35) -> (-5, -60) centre (-5, -35) ccw
  line L20 (-5, -60) -> (105, -60)
  arc A1 (105, -60) -> (130, -35) centre (105, -35) ccw
  line L21 (130, -35) -> (130, 100)
  line L22 (130, 100) -> (60, 100)
  line L23 (60, 100) -> (60, 70)
  line L24 (60, 70) -> (-25, 70)
  line L25 (-25, 70) -> (-25, 100)
  line L26 (-25, 100) -> (-30, 100)
  line L27 (-30, 100) -> (-30, -35)
  line L28 (98, -40) -> (0, -40)
  line L29 (0, -40) -> (0, 0)
  line L30 (0, 0) -> (98, 0)
  line L31 (98, 0) -> (98, -40)
  circle A2 centre (4, 30) radius 4
  circle A3 centre (94, 30) radius 4
  circle A4 centre (49, 30) radius 4
  circle A5 centre (19.5, 30) radius 4
  circle A6 centre (78.5, 30) radius 4
sketch "Sketch27" plane through (0, 0, 32) normal (0, 0, 1) x (-1, 0, 0)
  arc A0 (5, -60) -> (30, -35) centre (5, -35) ccw
  line L0 (30, -35) -> (30, 100)
  line L1 (30, 100) -> (-130, 100)
  line L2 (-130, 100) -> (-130, -35)
  arc A1 (-130, -35) -> (-105, -60) centre (-105, -35) ccw
  line L3 (-105, -60) -> (5, -60)
  line L4 (3, -58) -> (-103, -58)
  arc A2 (-128, -33) -> (-103, -58) centre (-103, -33) ccw
  line L5 (-128, -33) -> (-128, 98)
  line L6 (-128, 98) -> (28, 98)
  line L7 (28, 98) -> (28, -33)
  arc A3 (3, -58) -> (28, -33) centre (3, -33) ccw
extrude "Extrude42" add sketch "Sketch27" along normal blind 3 separate body contours A0 L0 L1 L2 A1 L3 | L4 A2 L5 L6 L7 A3 makes body 2
